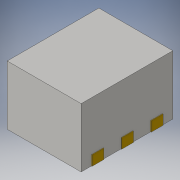
# Autodesk Inventor part: MC_TT240
Saved by Autodesk Inventor 2016 (Build 200138000, 138)
## iProperties
Created: 2016-08-30
Part Number: MC_TT240
Material: Generic
Document SubType Name: Modeling
Designer: jfixelle
Density: 1 g/cm^3
Appearance: Default
Author: jfixelle
Autodesk Inventor part; units mm, degrees
ref_plane "YZ Plane" through (0, 0, 0) normal (1, 0, 0) x (0, 1, 0)
ref_plane "XZ Plane" through (0, 0, 0) normal (0, 1, 0) x (-1, 0, 0)
ref_plane "XY Plane" through (0, 0, 0) normal (0, 0, 1) x (1, 0, 0)
sketch "Sketch1" plane through (0, 0, 0) normal (0, 1, 0) x (-1, 0, 0)
  line L0 (3.175, 3.935) -> (-3.175, 3.935)
  line L1 (-3.175, 3.935) -> (-3.175, -3.935)
  line L2 (-3.175, -3.935) -> (3.175, -3.935)
  line L3 (3.175, -3.935) -> (3.175, 3.935)
  point P0 (0, 0)
  dimension "d0" = 6.35
  dimension "d1" = 3.175
  dimension "d2" = 7.87
  dimension "d3" = 3.935
  constraints: 8 end point, 2 parallel, 1 horizontal, 1 perpendicular
  measures "d0" distance of L0.start L0.end
  measures "d1" distance from line of point (0, 0) L3
  measures "d2" distance of L2.end L0.start
  measures "d3" distance from line of point (0, 0) L2
extrude "Extrusion1" add sketch "Sketch1" along normal blind 5.08
sketch "Sketch2" plane through (0, 0, 0) normal (0, -1, 0) x (1, 0, 0)
  line L0 (3.225, 0.51) -> (1.955, 0.51)
  line L1 (1.955, 0.51) -> (1.955, -0.51)
  line L2 (1.955, -0.51) -> (3.225, -0.51)
  line L3 (3.225, -0.51) -> (3.225, 0.51)
  line L4 (3.175, 3.935) -> (3.175, -3.935) projected
  point P0 (0, 0)
  dimension "d6" = 1.02
  dimension "d7" = 0.51
  dimension "d8" = 0.05
  dimension "d9" = 1.27
  constraints: 8 end point, 2 parallel, 1 horizontal, 1 perpendicular
  measures "d6" distance of L2.end L0.start
  measures "d7" distance from line of point (0, 0) L0
  measures "d8" distance between parallel lines of L4 L3
  measures "d9" distance of L0.start L0.end
extrude "Extrusion2" add sketch "Sketch2" against normal blind 0.8467
pattern_linear "Rectangular Pattern1" count 3 spacing 2.54 along (0, 0, -1) of "Extrusion2" first direction both ways yes
mirror "Mirror1" about plane through (0, 0, 0) normal (1, 0, 0) of "Extrusion2", "Rectangular Pattern1"
body "Solid1"
